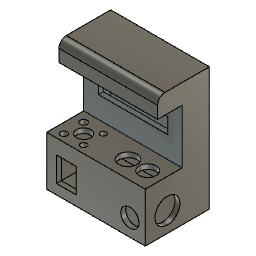
arcade_cabinet_1895 v9 (Autodesk Fusion 360 design; units mm, degrees)
Autodesk Fusion 360 part; units mm, degrees
box "BoxPrimitive1" add length 130 width 200 height 90 placed x (0, -1, 0) y (1, 0, 0) z (0, 0, 1) at (-80, 65, 0) in component "Body"
sketch "Sketch2" plane through (0, 0, 90) normal (0, 0, 1) x (-1, 0, 0) in component "Body"
  line L0 (80, 65) -> (-120, 65)
  line L1 (-120, 65) -> (-120, -65)
  line L2 (-120, -65) -> (80, -65)
  line L3 (80, -65) -> (80, 65)
  line L4 (70, 55) -> (-110, 55)
  line L5 (-110, 55) -> (-110, -55)
  line L6 (-110, -55) -> (70, -55)
  line L7 (70, -55) -> (70, 55)
  dimension "d6" = -10
extrude "Extrude1" cut sketch "Sketch2" against normal up to surface (80 mm away) contours L4 L5 L6 L7 in component "Body"
box "BoxPrimitive2" add length 55 width 200 height 80 placed x (0, -1, 0) y (1, 0, 0) z (0, 0, 1) at (-80, 65, 90) in component "Body"
sketch "Sketch4" plane through (0, 0, 170) normal (0, 0, 1) x (-1, 0, 0) in component "Body"
  line L0 (80, -10) -> (-120, -10)
  line L1 (-120, -10) -> (-120, -65)
  line L2 (-120, -65) -> (80, -65)
  line L3 (80, -65) -> (80, -10)
  line L4 (70, -20) -> (-110, -20)
  line L5 (-110, -20) -> (-110, -55)
  line L6 (-110, -55) -> (70, -55)
  line L7 (70, -55) -> (70, -20)
  dimension "d14" = -10
sketch "Sketch5" plane through (0, 10, 0) normal (0, -1, 0) x (1, 0, 0) in component "Body"
  line L0 (-80, 170) -> (-80, 90)
  line L1 (-80, 90) -> (-70, 90)
  line L2 (-70, 90) -> (110, 90)
  line L3 (110, 90) -> (120, 90)
  line L4 (120, 90) -> (120, 170)
  line L5 (120, 170) -> (-80, 170)
  line L6 (-57.5142, 112.4858) -> (97.5142, 112.4858)
  line L7 (97.5142, 112.4858) -> (97.5142, 147.5142)
  line L8 (97.5142, 147.5142) -> (-57.5142, 147.5142)
  line L9 (-57.5142, 147.5142) -> (-57.5142, 112.4858)
  dimension "d46" = -22.4858
extrude "Extrude2" cut sketch "Sketch4" against normal blind 90 contours L4 L5 L6 L7 in component "Body"
box "BoxPrimitive3" add length 75 width 200 height 10 placed x (0, -1, 0) y (1, 0, 0) z (0, 0, 1) at (-80, 10, 90) in component "Body"
sketch "Sketch7" plane through (0, 0, 0) normal (1, 0, 0) x (0, 1, 0) in component "Body"
sketch "Sketch8" plane through (0, 0, 100) normal (0, 0, 1) x (-1, 0, 0) in component "Body"
  line L0 (80, 65) -> (-120, 65)
  line L1 (-120, 65) -> (-120, -10)
  line L2 (-120, -10) -> (80, -10)
  line L3 (80, -10) -> (80, 65)
  circle A0 centre (38.5156, 25.2185) radius 33.0643
  circle A1 centre (-50, 30) radius 18.3816
  circle A2 centre (-90, 30) radius 17.1816
extrude "Extrude3" cut sketch "Sketch8" against normal blind 30 contours A0 | A1 | A2 in component "Body"
sketch "Sketch9" plane through (0, -65, 0) normal (0, -1, 0) x (1, 0, 0) in component "Body"
  line L0 (-80, 100) -> (-80, 0)
  line L1 (-80, 0) -> (120, 0)
  line L2 (120, 0) -> (120, 100)
  line L3 (120, 100) -> (-80, 100)
  circle A0 centre (88.8722, 34.3956) radius 18.5203
box "BoxPrimitive4" cut length 50 width 40 height -40 placed x (0, 0, 1) y (-1, 0, 0) z (0, -1, 0) at (-20, -65, 20) in component "Body"
extrude "Extrude4" cut sketch "Sketch9" against normal blind 30 contours A0 in component "Body"
sketch "Sketch10" plane through (120, 0, 0) normal (1, 0, 0) x (0, 1, 0) in component "Body"
  line L0 (-65, 100) -> (-65, 0)
  line L1 (-65, 0) -> (65, 0)
  line L2 (65, 0) -> (65, 170)
  line L3 (65, 170) -> (10, 170)
  line L4 (10, 170) -> (10, 100)
  line L5 (10, 100) -> (-65, 100)
  circle A0 centre (-20, 40) radius 25.364
extrude "Extrude5" cut sketch "Sketch10" against normal blind 30 contours A0 in component "Body"
box "BoxPrimitive5" cut length 20 width 10 height -10 placed x (0, 0, 1) y (1, 0, 0) z (0, 1, 0) at (90, 65, 20) in component "Body"
box "BoxPrimitive6" add length 105 width 200 height 80 placed x (0, -1, 0) y (1, 0, 0) z (0, 0, 1) at (-80, 65, 170) in component "Body"
fillet "Fillet1" radius 15 1 edges at (20, -40, 250) in component "Body"
delete_face "DeleteFace1" 1 faces at (-27.9196, -56.539, 86.6667) in component "Body"
sketch "Sketch13" plane through (0, 0, 100) normal (0, 0, 1) x (-1, 0, 0) in component "Body"
  circle A0 centre (-90, 30) radius 17.1816
  circle A1 centre (-50, 30) radius 18.3816
  line L0 (-120, 65) -> (-120, -10)
  line L1 (-120, -10) -> (80, -10)
  line L2 (80, -10) -> (80, 65)
  line L3 (80, 65) -> (-120, 65)
  circle A2 centre (40, 30) radius 14.4729
  circle A3 centre (60, 50) radius 6.8219
  circle A4 centre (20, 50) radius 6.137
  circle A5 centre (20, 10) radius 6.0263
  circle A6 centre (60, 10) radius 7.3219
  point P0 (60, 50)
extrude "Extrude7" cut sketch "Sketch13" against normal blind 20 contours A2 | A3 | A4 | A5 | A6 in component "Body"
move_face "OffsetFaces1" offset -40 1 faces at (53.3333, -6.6667, 170) in component "Body"
sketch "Sketch1" plane through (0, 10, 0) normal (0, -1, 0) x (1, 0, 0)
  line L0 (-80, 100) -> (120, 100)
  line L1 (120, 100) -> (120, 210)
  line L2 (120, 210) -> (-80, 210)
  line L3 (-80, 210) -> (-80, 100)
box "BoxPrimitive7" cut length 31.2354 width 140.7967 height -45 placed x (0, 0, 1) y (-1, 0, 0) z (0, -1, 0) at (90.7967, 10, 143.7646) in component "Body"
component "Body" placed x (1, 0, 0) y (0, 1, 0) z (0, 0, 1) at (0, 0, 0)
